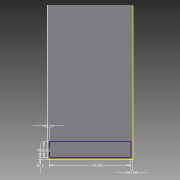
# Autodesk Inventor part: base-frame
Saved by Autodesk Inventor 2015 (Build 190159000, 159)
## iProperties
Created: 2014-07-15
Part Number: base-frame
Material: Generic
Document SubType Name: Modeling
Designer: pc
Density: 1 g/cm^3
Appearance: Default
Author: pc
Autodesk Inventor part; units mm, degrees
ref_plane "YZ Plane" through (0, 0, 0) normal (1, 0, 0) x (0, 1, 0)
ref_plane "XZ Plane" through (0, 0, 0) normal (0, 1, 0) x (-1, 0, 0)
ref_plane "XY Plane" through (0, 0, 0) normal (0, 0, 1) x (1, 0, 0)
sketch "Sketch1" plane through (0, 0, 0) normal (0, 1, 0) x (-1, 0, 0)
  line L0 (0, 0) -> (79.12, 0)
  line L1 (79.12, 0) -> (79.12, -44)
  line L2 (79.12, -44) -> (0, -44)
  line L3 (0, -44) -> (0, 0)
  dimension "d0" = 44
  dimension "d1" = 79.12
  constraints: 8 end point, 2 parallel, 1 horizontal, 1 perpendicular
  measures "d0" distance of L2.end L0.start
  measures "d1" distance of L0.start L0.end
extrude "Extrusion1" add sketch "Sketch1" along normal blind 6
sketch "Sketch2" plane through (0, 6, 0) normal (0, 1, 0) x (1, 0, 0)
  line L0 (-9.12, 1) -> (-1, 1)
  line L1 (-1, 1) -> (-1, 43)
  line L2 (-1, 43) -> (-9.12, 43)
  line L3 (-9.12, 43) -> (-9.12, 1)
  line L4 (0, 0) -> (0, 44) projected
  line L5 (-79.12, 0) -> (0, 0) projected
  line L6 (0, 44) -> (-79.12, 44) projected
  dimension "d4" = 42
  dimension "d5" = 8.12
  dimension "d9" = 1
  dimension "d10" = 1
  dimension "d12" = 1
  constraints: 8 end point, 2 parallel, 1 horizontal, 1 perpendicular
  measures "d4" distance of L0.end L1.end
  measures "d5" distance of L0.start L0.end
  measures "d9" distance between parallel lines of L0 L5
  measures "d10" distance between parallel lines of L6 L2
  measures "d12" distance between parallel lines of L4 L1
equation "\"d0\" = basew"
equation "\"d1\" = baseh"
equation "\"d2\" = base_thick"
equation "\"d4\" = wallw"
equation "\"d5\" = wall1slot"
equation "\"d9\" = -0.5 * wallw + 0.5 * basew"
equation "\"d12\" = 0.5 * baseextra"
equation "\"printer3dtolerance\" = 0.12"
equation "\"wallw\" = 42"
equation "\"wallh\" = 44"
equation "\"cornerrad\" = 2"
equation "\"baseextra\" = 2"
equation "\"wall1_thick\" = 8"
equation "\"wall2_thick\" = 6.4"
equation "\"wall3_thick\" = 4"
equation "\"wall1slot\" = 8.12"
equation "\"wall2slot\" = 6.52"
equation "\"wall3slot\" = 4.12"
equation "\"gap2\" = 28"
equation "\"baseh\" = 79.12"
equation "\"basew\" = 44"
equation "\"base_thick\" = 6"
equation "\"base_slots_depth\" = 4"
body "Solid1"
